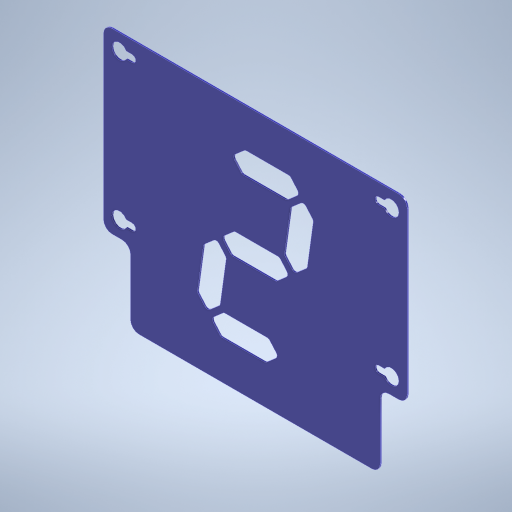
# Autodesk Inventor part: TorsoColorMarker
Saved by Autodesk Inventor 2024.2 (Build 282272000, 272)
## iProperties
Created: 2024-01-22
Part Number: TorsoColorMarker
Material: Polypropylene
Document SubType Name: Modeling
Designer: Masato Kubotera
Density: 0.899 g/cm^3
Appearance: Smooth - Navy
Mass: 15.4158 g
Surface Area: 466.542 cm^2
Volume: 17.1477 cm^3
Author: Masato Kubotera
Autodesk Inventor part; units mm, degrees
ref_plane "YZ Plane" through (0, 0, 0) normal (1, 0, 0) x (0, 1, 0)
ref_plane "XZ Plane" through (0, 0, 0) normal (0, 1, 0) x (-1, 0, 0)
ref_plane "XY Plane" through (0, 0, 0) normal (0, 0, 1) x (1, 0, 0)
derived "TorsoCoverFrameBasis.ipt"
sketch "Sketch1" plane through (0, 0, 0) normal (1, 0, 0) x (0, 1, 0)
  line L0 (-90, 74.5) -> (90, 74.5)
  line L1 (90, 74.5) -> (90, -74.5)
  line L2 (90, -74.5) -> (-90, -74.5)
  line L3 (-90, -74.5) -> (-90, 74.5)
  line L4 (-90, 74.5) -> (90, -74.5) construction
  line L5 (90, 74.5) -> (-90, -74.5) construction
  line L6 (85, 74.5) -> (85, 46.75)
  line L7 (85, 46.75) -> (90, 46.75)
  line L8 (0, 74.5) -> (0, -74.5)
  line L9 (90, 0) -> (-90, 0) construction
  arc A0 (85, 49.75) -> (85, 46.75) centre (85, 48.25) ccw
  line L10 (-90, 74.5) -> (-90, -74.5)
  circle A1 centre (73, 65) radius 3 construction
  arc A2 (73, 67.1) -> (73, 62.9) centre (73, 65) ccw construction
  line L11 (73, 67.1) -> (76.5201, 67.1) construction
  arc A3 (76.5201, 62.9) -> (76.5201, 67.1) centre (80.5, 65) ccw construction
  line L12 (73, 65) -> (80.5, 65) construction
  line L13 (73, 62.9) -> (76.5201, 62.9) construction
  line L14 (90, 28.75) -> (85, 28.75) construction
  line L15 (90, 14.75) -> (85, 14.75) construction
  line L16 (90, 21.75) -> (85, 21.75) construction
  arc A4 (85, -3.25) -> (85, -6.25) centre (85, -4.75) ccw
  line L17 (85, -3.25) -> (90, -3.25)
  line L18 (85, -6.25) -> (85, -74.5)
  line L19 (90, -31) -> (-90, -31)
  line L20 (74, -31) -> (74, -74.5)
  line L21 (-90, 21.75) -> (90, 21.75) construction
  line L22 (73, -19.4) -> (76.5201, -19.4) construction
  line L23 (73, -21.5) -> (80.5, -21.5) construction
  line L24 (73, -23.6) -> (76.5201, -23.6) construction
  arc A5 (73, -19.4) -> (73, -23.6) centre (73, -21.5) ccw construction
  circle A6 centre (73, -21.5) radius 3 construction
  arc A7 (76.5201, -23.6) -> (76.5201, -19.4) centre (80.5, -21.5) ccw construction
  arc A8 (74, -31) -> (74, -34) centre (74, -32.5) ccw
  point P0 (0, 0)
  point P1 (85, -74.5)
  point P2 (85, 65)
  point P3 (85, -21.5)
sketch "Sketch2" plane through (0, 0, 0) normal (1, 0, 0) x (0, 1, 0)
  arc A0 (17.3504, 10.1935) -> (17.8216, 8.603) centre (19.331, 9.9151) ccw
  line L0 (21.7067, 4.1337) -> (17.8216, 8.603)
  arc A1 (14.8027, 5.9788) -> (13.2933, 6.6667) centre (13.2933, 4.6667) ccw
  line L1 (14.8027, 5.9788) -> (18.6879, 1.5094)
  arc A2 (-18.4906, 1.3121) -> (-18.6879, -1.5094) centre (-17.1785, -0.1973) ccw
  line L2 (-12.8952, 6.1761) -> (-18.4906, 1.3121)
  arc A3 (-11.5831, 6.6667) -> (-12.8952, 6.1761) centre (-11.5831, 4.6667) ccw
  line L3 (-18.6879, -1.5094) -> (-14.8027, -5.9788)
  line L4 (-21.481, -36.0589) -> (-27.0763, -40.9228)
  arc A4 (-29.8979, -40.7255) -> (-27.0763, -40.9228) centre (-28.3885, -39.4134) ccw
  line L5 (-29.8979, -40.7255) -> (-33.783, -36.2562)
  arc A5 (-34.2542, -34.6657) -> (-33.783, -36.2562) centre (-32.2736, -34.9441) ccw
  line L6 (-17.3504, -10.1935) -> (-20.8126, -34.8278)
  arc A6 (-17.3504, -10.1935) -> (-17.8216, -8.603) centre (-19.331, -9.9151) ccw
  line L7 (-30.792, -10.0314) -> (-34.2542, -34.6657)
  arc A7 (-21.481, -36.0589) -> (-20.8126, -34.8278) centre (-22.7931, -34.5495) ccw
  line L8 (-21.7067, -4.1337) -> (-17.8216, -8.603)
  arc A8 (-30.1236, -8.8003) -> (-30.792, -10.0314) centre (-28.8115, -10.3097) ccw
  arc A9 (-21.7067, -4.1337) -> (-24.5283, -3.9364) centre (-23.2161, -5.4458) ccw
  line L9 (-24.5283, -3.9364) -> (-30.1236, -8.8003)
  arc A10 (-17.8877, -38.1925) -> (-19.1998, -38.6831) centre (-17.8877, -40.1925) ccw
  arc A11 (21.481, 36.0589) -> (20.8126, 34.8278) centre (22.7931, 34.5495) ccw
  line L10 (20.8126, 34.8278) -> (17.3504, 10.1935)
  line L11 (29.8979, 40.7255) -> (33.783, 36.2562)
  line L12 (27.0763, 40.9228) -> (21.481, 36.0589)
  arc A12 (29.8979, 40.7255) -> (27.0763, 40.9228) centre (28.3885, 39.4134) ccw
  arc A13 (21.1073, 50.838) -> (19.5979, 51.5259) centre (19.5979, 49.5259) ccw
  arc A14 (17.8877, 38.1925) -> (19.1998, 38.6831) centre (17.8877, 40.1925) ccw
  line L13 (21.1073, 50.838) -> (24.9924, 46.3686)
  arc A15 (24.7951, 43.5471) -> (24.9924, 46.3686) centre (23.483, 45.0565) ccw
  line L14 (19.1998, 38.6831) -> (24.7951, 43.5471)
  line L15 (-23.5933, 4.1337) -> (-27.4785, 8.603)
  line L16 (-24.4875, 34.8278) -> (-27.9496, 10.1935)
  arc A16 (-27.9496, 10.1935) -> (-27.4785, 8.603) centre (-25.9691, 9.9151) ccw
  line L17 (-15.4022, 40.7255) -> (-11.517, 36.2562)
  line L18 (-11.0459, 34.6657) -> (-14.508, 10.0314)
  line L19 (-16.7143, 42.235) -> (-22.2812, 2.6242) construction
  arc A17 (-15.1764, 8.8003) -> (-14.508, 10.0314) centre (-16.4886, 10.3097) ccw
  line L20 (-15.1764, 8.8003) -> (-20.7718, 3.9364)
  arc A18 (-23.5933, 4.1337) -> (-20.7718, 3.9364) centre (-22.0839, 5.4458) ccw
  line L21 (-6.9888, 38.1925) -> (17.8877, 38.1925)
  line L22 (26.3045, 44.8592) -> (-13.6955, 44.8592) construction
  line L23 (-5.2786, 51.5259) -> (19.5979, 51.5259)
  arc A19 (-8.4982, 38.8804) -> (-6.9888, 38.1925) centre (-6.9888, 40.1925) ccw
  arc A20 (-12.186, 46.1713) -> (-12.3833, 43.3498) centre (-10.8739, 44.6619) ccw
  line L24 (-6.5907, 51.0353) -> (-12.186, 46.1713)
  arc A21 (-5.2786, 51.5259) -> (-6.5907, 51.0353) centre (-5.2786, 49.5259) ccw
  arc A22 (-11.0459, 34.6657) -> (-11.517, 36.2562) centre (-13.0264, 34.9441) ccw
  arc A23 (-15.4022, 40.7255) -> (-18.2237, 40.9228) centre (-16.9116, 39.4134) ccw
  line L25 (-18.2237, 40.9228) -> (-23.8191, 36.0589)
  arc A24 (-23.8191, 36.0589) -> (-24.4875, 34.8278) centre (-22.5069, 34.5495) ccw
  line L26 (-12.3833, 43.3498) -> (-8.4982, 38.8804)
  line L27 (-13.2933, -6.6667) -> (11.5831, -6.6667)
  arc A25 (15.1764, -8.8003) -> (14.508, -10.0314) centre (16.4886, -10.3097) ccw
  line L28 (14.508, -10.0314) -> (11.0459, -34.6657)
  arc A26 (8.4982, -38.8804) -> (6.9888, -38.1925) centre (6.9888, -40.1925) ccw
  line L29 (-17.8877, -38.1925) -> (6.9888, -38.1925)
  line L30 (-19.1998, -38.6831) -> (-24.7951, -43.5471)
  arc A27 (-24.7951, -43.5471) -> (-24.9924, -46.3686) centre (-23.483, -45.0565) ccw
  line L31 (-19.5979, -51.5259) -> (5.2786, -51.5259)
  arc A28 (27.9496, -10.1935) -> (27.4785, -8.603) centre (25.9691, -9.9151) ccw
  line L32 (27.9496, -10.1935) -> (24.4875, -34.8278)
  arc A29 (23.5933, -4.1337) -> (20.7718, -3.9364) centre (22.0839, -5.4458) ccw
  arc A30 (11.0459, -34.6657) -> (11.517, -36.2562) centre (13.0264, -34.9441) ccw
  line L33 (6.5907, -51.0353) -> (12.186, -46.1713)
  arc A31 (12.186, -46.1713) -> (12.3833, -43.3498) centre (10.8739, -44.6619) ccw
  line L34 (34.2542, 34.6657) -> (30.792, 10.0314)
  arc A32 (34.2542, 34.6657) -> (33.783, 36.2562) centre (32.2736, 34.9441) ccw
  arc A33 (30.1236, 8.8003) -> (30.792, 10.0314) centre (28.8115, 10.3097) ccw
  line L35 (30.1236, 8.8003) -> (24.5283, 3.9364)
  arc A34 (21.7067, 4.1337) -> (24.5283, 3.9364) centre (23.2161, 5.4458) ccw
  line L36 (8.4982, -38.8804) -> (12.3833, -43.3498)
  line L37 (15.4022, -40.7255) -> (11.517, -36.2562)
  arc A35 (15.4022, -40.7255) -> (18.2237, -40.9228) centre (16.9116, -39.4134) ccw
  line L38 (23.5933, -4.1337) -> (27.4785, -8.603)
  arc A36 (23.8191, -36.0589) -> (24.4875, -34.8278) centre (22.5069, -34.5495) ccw
  line L39 (23.8191, -36.0589) -> (18.2237, -40.9228)
  arc A37 (5.2786, -51.5259) -> (6.5907, -51.0353) centre (5.2786, -49.5259) ccw
  line L40 (20.7718, -3.9364) -> (15.1764, -8.8003)
  line L41 (12.8952, -6.1761) -> (18.4906, -1.3121)
  arc A38 (18.4906, -1.3121) -> (18.6879, 1.5094) centre (17.1785, 0.1973) ccw
  arc A39 (11.5831, -6.6667) -> (12.8952, -6.1761) centre (11.5831, -4.6667) ccw
  arc A40 (-21.1073, -50.838) -> (-19.5979, -51.5259) centre (-19.5979, -49.5259) ccw
  arc A41 (-14.8027, -5.9788) -> (-13.2933, -6.6667) centre (-13.2933, -4.6667) ccw
  line L42 (-24.9924, -46.3686) -> (-21.1073, -50.838)
  line L43 (0.8551, 6.6667) -> (-0.8551, -6.6667) construction
  line L44 (-11.5831, 6.6667) -> (13.2933, 6.6667)
  line L45 (0, 74.5) -> (0, -74.5) construction
  line L46 (-90, 74.5) -> (90, 74.5) projected
  line L47 (90, -74.5) -> (-90, -74.5) projected
  line L48 (90, 74.5) -> (90, -74.5) projected
  arc A42 (76.5201, 62.9) -> (76.5201, 67.1) centre (80.5, 65) ccw projected
  line L49 (73, 67.1) -> (76.5201, 67.1) projected
  arc A43 (73, 67.1) -> (73, 62.9) centre (73, 65) ccw projected
  line L50 (73, 62.9) -> (76.5201, 62.9) projected
  line L51 (-90, 0) -> (90, 0) construction
  arc A44 (76.5201, -23.6) -> (76.5201, -19.4) centre (80.5, -21.5) ccw projected
  line L52 (73, -19.4) -> (76.5201, -19.4) projected
  arc A45 (73, -19.4) -> (73, -23.6) centre (73, -21.5) ccw projected
  line L53 (73, -23.6) -> (76.5201, -23.6) projected
  arc A46 (-76.5201, 67.1) -> (-76.5201, 62.9) centre (-80.5, 65) ccw
  line L54 (-73, 67.1) -> (-76.5201, 67.1)
  arc A47 (-73, 62.9) -> (-73, 67.1) centre (-73, 65) ccw
  line L55 (-73, 62.9) -> (-76.5201, 62.9)
  arc A48 (-76.5201, -19.4) -> (-76.5201, -23.6) centre (-80.5, -21.5) ccw
  line L56 (-73, -19.4) -> (-76.5201, -19.4)
  arc A49 (-73, -23.6) -> (-73, -19.4) centre (-73, -21.5) ccw
  line L57 (-73, -23.6) -> (-76.5201, -23.6)
  line L58 (-90, 74.5) -> (-90, -74.5)
  line L59 (90, -31) -> (-90, -31) projected
  line L60 (74, -31) -> (74, -74.5) projected
  line L61 (-90, -31) -> (90, -31)
  line L62 (-74, -31) -> (-74, -74.5)
  point P0 (0, 0)
  point P1 (17.2236, 9.2909)
  point P2 (23.0188, 2.6242)
  point P3 (14.2048, 6.6667)
  point P4 (20, 0)
  point P5 (-12.3309, 6.6667)
  point P6 (-20, 0)
  point P7 (-14.2048, -6.6667)
  point P8 (-20.9166, -35.5683)
  point P9 (-28.5858, -42.235)
  point P10 (-34.381, -35.5683)
  point P11 (-17.2236, -9.2909)
  point P12 (-30.688, -9.2909)
  point P13 (-18.6354, -38.1925)
  point P14 (-23.0188, -2.6242)
  point P15 (20.9166, 35.5683)
  point P16 (28.5858, 42.235)
  point P17 (34.381, 35.5683)
  point P18 (20.5093, 51.5259)
  point P19 (18.6354, 38.1925)
  point P20 (-28.0765, 9.2909)
  point P21 (-24.3834, 35.5683)
  point P22 (-10.919, 35.5683)
  point P23 (-7.9002, 38.1925)
  point P24 (-14.6121, 9.2909)
  point P25 (-6.0263, 51.5259)
  point P26 (12.3309, -6.6667)
  point P27 (14.6121, -9.2909)
  point P28 (10.919, -35.5683)
  point P29 (7.9002, -38.1925)
  point P30 (-26.3045, -44.8592)
  point P31 (6.0263, -51.5259)
  point P32 (-20.5093, -51.5259)
  point P33 (22.2812, -2.6242)
  point P34 (28.0765, -9.2909)
  point P35 (24.3834, -35.5683)
  point P36 (13.6955, -44.8592)
  point P37 (30.688, 9.2909)
  point P38 (16.7143, -42.235)
  point P39 (0, 0)
  point P40 (0, 0)
  point P41 (11.5611, -31)
  point P42 (25.0254, -31)
  dimension "d9" = 4
  dimension "d10" = 13.3333
  dimension "d11" = 13.3333
  dimension "d12" = 40
  dimension "d13" = 40
  dimension "d14" = 2
  dimension "d16" = 45.3
  dimension "d17" = 45.3
  dimension "d18" = 45.3
  dimension "d21" = 8
  dimension "d29" = 0
  constraints: 106 end point, 92 point on circle, 84 point on line, 46 centre point, 24 tangent, 17 symmetric about line, 11 equal radius, 7 midpoint, 5 collinear, 5 parallel, 3 horizontal, 1 perpendicular, 189 other
  measures "d9" distance between parallel lines of L17 L26
  measures "d10" distance between parallel lines of L21 L23
  measures "d11" distance between parallel lines of L18 L16
  measures "d12" distance of L22.start L22.end
  measures "d13" distance of L19.start L19.end
  measures "d14" radius of A23
  measures "d16" distance of L17.start L11.start
  measures "d17" distance of L17.start L8.start
  measures "d18" distance of L23.start L44.start
  measures "d21" angle of L10 L45
  measures "d29" distance from line of point (0, 0) L45
extrude "Extrusion1" add sketch "Sketch2" along normal blind 0.75 contours A7 L6 L59 L28 A30 L37 A35 L39 A36 L32 L60 L47 L62 L7 A5 L5 A4 L4 | L6 A6 L8 A9 L9 A8 L7 L59 L58 L46 L48 L32 A28 L38 A29 L40 A25 L28 | L59 L32 A36 L39 A35 L37 A30 L28 | L28 A25 L40 A29 L38 A28 L32 L59 | L15 A16 L16 A24 L25 A23 L17 A22 L18 A17 L20 A18
fillet "R5" radius 5 8 edges at (0.375, -90, 74.5) (0.375, 90, 74.5) (0.375, 90, -31) (0.375, 74, -74.5) (0.375, -90, -31) (0.375, -74, -31) (0.375, -74, -74.5) (0.375, 74, -31)
equation "\"d11\" = d10"
equation "\"d13\" = d12"
body "Solid1"
